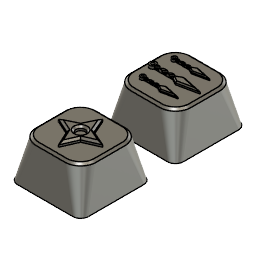
Ninjakeys (Autodesk Fusion 360 design; units mm, degrees)
part number: 2026-03-30-17-35-38-654
Autodesk Fusion 360 part; units mm, degrees
note: some values were not read from the file. Chosen so that the rebuilt part matches the saved one: which face or edge a step refers to.
sketch "Sketch1" plane through (0, 0, 0) normal (0, 1, 0) x (1, 0, 0)
  line L0 (7, -9) -> (-7, -9)
  line L1 (-9, -7) -> (-9, 7)
  line L2 (-7, 9) -> (7, 9)
  line L3 (9, 7) -> (9, -7)
  line L4 (9, -9) -> (-9, 9) construction
  line L5 (-9, -9) -> (9, 9) construction
  arc A0 (-7, 9) -> (-9, 7) centre (-7, 7) ccw
  arc A1 (9, 7) -> (7, 9) centre (7, 7) ccw
  arc A2 (7, -9) -> (9, -7) centre (7, -7) ccw
  arc A3 (-9, -7) -> (-7, -9) centre (-7, -7) ccw
  dimension "d1" = 18
  dimension "d2" = 18
  dimension "d3" = 2
  dimension "d4" = 2
  dimension "d5" = 2
  dimension "d6" = 2
  constraint horizontal L0
  constraint perpendicular L0 L1
  constraint parallel L0 L2
  constraint parallel L1 L3
  constraint coincident L4 origin
  constraint coincident L5 origin
  constraint coincident L4.end L2
  constraint coincident L4.end L1
  constraint tangent L2 A0
  constraint tangent L1 A0
  constraint coincident L5.end L2
  constraint coincident L5.end L3
  constraint tangent L2 A1
  constraint tangent L3 A1
  constraint coincident L4.start L0
  constraint coincident L4.start L3
  constraint tangent L0 A2
  constraint tangent L3 A2
  constraint coincident L5.start L0
  constraint coincident L5.start L1
  constraint tangent L0 A3
  constraint tangent L1 A3
  measures "d1" distance of L4.end L5.end
  measures "d2" distance of L5.start L4.end
  measures "d3" radius of A0
  measures "d4" radius of A1
  measures "d5" radius of A2
  measures "d6" radius of A3
ref_plane "WorkPlane1" through (0, 10, 0) normal (0, 1, 0) x (1, 0, 0)
sketch "Sketch2" plane through (0, 10, 0) normal (0, 1, 0) x (1, 0, 0)
  line L0 (3.5, -7.5) -> (-3.5, -7.5)
  line L1 (-7.5, -3.5) -> (-7.5, 3.5)
  line L2 (-3.5, 7.5) -> (3.5, 7.5)
  line L3 (7.5, 3.5) -> (7.5, -3.5)
  line L4 (7.5, -7.5) -> (-7.5, 7.5) construction
  line L5 (-7.5, -7.5) -> (7.5, 7.5) construction
  arc A0 (-3.5, 7.5) -> (-7.5, 3.5) centre (-3.5, 3.5) ccw
  arc A1 (-7.5, -3.5) -> (-3.5, -7.5) centre (-3.5, -3.5) ccw
  arc A2 (7.5, 3.5) -> (3.5, 7.5) centre (3.5, 3.5) ccw
  arc A3 (3.5, -7.5) -> (7.5, -3.5) centre (3.5, -3.5) ccw
  dimension "d8" = 15
  dimension "d9" = 15
  dimension "d10" = 4
  dimension "d11" = 4
  dimension "d12" = 4
  dimension "d13" = 4
  constraint horizontal L0
  constraint perpendicular L0 L1
  constraint parallel L0 L2
  constraint parallel L1 L3
  constraint coincident L4 origin
  constraint coincident L5 origin
  constraint coincident L4.end L2
  constraint coincident L4.end L1
  constraint tangent L2 A0
  constraint tangent L1 A0
  constraint coincident L5.start L0
  constraint coincident L5.start L1
  constraint tangent L0 A1
  constraint tangent L1 A1
  constraint coincident L5.end L2
  constraint coincident L5.end L3
  constraint tangent L2 A2
  constraint tangent L3 A2
  constraint coincident L4.start L0
  constraint coincident L4.start L3
  constraint tangent L0 A3
  constraint tangent L3 A3
  measures "d8" distance of L4.end L5.end
  measures "d9" distance of L5.start L4.end
  measures "d10" radius of A0
  measures "d11" radius of A1
  measures "d12" radius of A2
  measures "d13" radius of A3
loft "Loft1" add profiles "Sketch1", "Sketch2" section 1 section 2 makes body 1
shell "Shell1" thickness 1 removed faces 1 at (2.3333, 0, 3) on bodies 1
sketch "Sketch4" plane through (0, 9, 0) normal (0, -1, 0) x (1, 0, 0)
  spline S0 degree 3 poles (-3.7981, -6.6388) (-3.9185, -6.6384) (-4.2445, -6.6305) (-4.797, -6.4579) (-4.9562, -6.3904) (-5.4554, -6.1276) (-5.7528, -5.8783) (-6.2352, -5.2918) (-6.4106, -4.9558) (-6.643, -4.1949) (-6.6388, -3.8753) (-6.6388, -2.5029) (-6.6388, -1.6238) (-6.6388, 0.4704) (-6.6388, 1.6711) (-6.6388, 3.2353) (-6.6592, 3.6248) (-6.6079, 4.3124) (-6.5325, 4.6087) (-6.2807, 5.2077) (-6.0878, 5.496) (-5.5896, 6.0247) (-5.2732, 6.2437) (-4.6118, 6.5389) (-4.274, 6.617) (-3.6622, 6.6501) (-3.39, 6.6388) (-2.7262, 6.6388) (-2.3393, 6.6388) (-1.2893, 6.6388) (-0.6369, 6.6388) (1.3044, 6.6388) (2.5692, 6.6388) (3.8951, 6.6388) (4.224, 6.6347) (4.783, 6.4632) (4.9424, 6.3967) (5.4429, 6.1366) (5.7418, 5.8887) (6.2275, 5.3043) (6.4047, 4.9689) (6.6432, 4.2018) (6.6388, 3.8836) (6.6388, 3.4954) (6.6388, 3.373) (6.6388, 1.3089) (6.6388, -0.5696) (6.6388, -2.8908) (6.6471, -3.377) (6.6368, -3.9301) (6.6315, -4.0102) (6.5893, -4.4056) (6.5019, -4.705) (6.2091, -5.3351) (5.9762, -5.6431) (5.4143, -6.1554) (5.0851, -6.3487) (4.3595, -6.61) (4.0322, -6.6388) (2.4883, -6.6388) (1.2237, -6.6388) (0, -6.6388) (-1.2622, -6.6388) (-2.5245, -6.6388) (-3.7902, -6.6388) (-3.794, -6.6388) (-3.7981, -6.6388) knots -2.01973615 -2.01973615 -2.01973615 -2.01973615 -1.98778124 -1.98778124 -1.9735129 -1.9735129 -1.93956421 -1.93956421 -1.90404512 -1.90404512 -1.86164762 -1.86164762 -1.7780832 -1.7780832 -1.65590778 -1.65590778 -1.61360327 -1.61360327 -1.57829605 -1.57829605 -1.53554689 -1.53554689 -1.48489072 -1.48489072 -1.43585563 -1.43585563 -1.39416826 -1.39416826 -1.33065911 -1.33065911 -1.21603599 -1.21603599 -0.97815888 -0.97815888 -0.95834343 -0.95834343 -0.94963949 -0.94963949 -0.92889287 -0.92889287 -0.90717906 -0.90717906 -0.88083394 -0.88083394 -0.86805791 -0.86805791 -0.65819989 -0.65819989 -0.60006747 -0.60006747 -0.58983944 -0.58983944 -0.54756375 -0.54756375 -0.49178961 -0.49178961 -0.43273454 -0.43273454 -0.36711002 -0.36711002 0 0 0 0.37866803 0.37866803 0.37973785 0.37973785 0.37973785 0.37973785
  circle A0 centre (0, 0) radius 2.75
  line L0 (2, -0.585) -> (-2, -0.585)
  line L1 (-2, -0.585) -> (-2, 0.585)
  line L2 (-2, 0.585) -> (2, 0.585)
  line L3 (2, 0.585) -> (2, -0.585)
  line L4 (2, -0.585) -> (-2, 0.585) construction
  line L5 (-2, -0.585) -> (2, 0.585) construction
  line L6 (0.585, -2) -> (-0.585, -2)
  line L7 (-0.585, -2) -> (-0.585, 2)
  line L8 (-0.585, 2) -> (0.585, 2)
  line L9 (0.585, 2) -> (0.585, -2)
  line L10 (0.585, -2) -> (-0.585, 2) construction
  line L11 (-0.585, -2) -> (0.585, 2) construction
  dimension "d15" = 5.5
  dimension "d16" = 4
  dimension "d17" = 1.17
  dimension "d18" = 1.17
  dimension "d19" = 4
  constraint coincident A0.centre origin
  constraint horizontal L0
  constraint perpendicular L0 L1
  constraint parallel L0 L2
  constraint parallel L1 L3
  constraint coincident L4 A0.centre
  constraint coincident L5 A0.centre
  constraint horizontal L6
  constraint perpendicular L6 L7
  constraint parallel L6 L8
  constraint parallel L7 L9
  constraint coincident L10 A0.centre
  constraint coincident L11 A0.centre
  measures "d15" diameter of A0
  measures "d16" distance of L1.end L2.end
  measures "d17" distance of L0.end L1.end
  measures "d18" distance of L7.end L8.end
  measures "d19" distance of L6.end L7.end
extrude "Extrude1" add sketch "Sketch4" along normal blind 6 contours A0 bodies 1
chamfer "Chamfer1" distance 0.5 angle 45 8 edges at (0, 10, 7.5) (6.3284, 10, 6.3284) (7.5, 10, 0) (6.3284, 10, -6.3284) (0, 10, -7.5) (-6.3284, 10, -6.3284) (-7.5, 10, 0) (-6.3284, 10, 6.3284) on bodies 1
sketch "Sketch5" plane through (0, 10, 0) normal (0, 1, 0) x (-1, 0, 0)
  spline S0 degree 3 poles (3.5, -7) (2.6099, -7) (1.7198, -7) (0.1872, -7) (-0.4553, -7) (-1.5919, -7) (-2.0861, -7) (-2.8868, -7) (-3.1934, -7) (-3.5, -7) (-3.7493, -7) (-4.1606, -6.971) (-5.0783, -6.6613) (-5.5771, -6.3727) (-6.3727, -5.5771) (-6.6613, -5.0783) (-6.971, -4.1606) (-7, -3.7493) (-7, -3.5) (-7, -2.6136) (-7, -1.7272) (-7, -0.1967) (-7, 0.4474) (-7, 1.587) (-7, 2.0824) (-7, 2.8853) (-7, 3.1926) (-7, 3.5) (-7, 3.7493) (-6.971, 4.1606) (-6.6613, 5.0783) (-6.3727, 5.5771) (-5.5771, 6.3727) (-5.0783, 6.6613) (-4.1606, 6.971) (-3.7493, 7) (-3.5, 7) (-2.5733, 7) (-1.6466, 7) (-0.0937, 7) (0.5324, 7) (1.6403, 7) (2.1219, 7) (2.9024, 7) (3.2012, 7) (3.5, 7) (3.7493, 7) (4.1606, 6.971) (5.0782, 6.6613) (5.577, 6.3727) (6.3727, 5.5771) (6.6612, 5.0783) (6.971, 4.1607) (7, 3.7493) (7, 3.5) (7, 2.7834) (7, 2.0667) (7, 0.8078) (7, 0.2654) (7, -0.694) (7, -1.1112) (7, -1.8493) (7, -2.1702) (7, -2.7379) (7, -2.9848) (7, -3.3211) (7, -3.4105) (7, -3.5) (7, -3.6826) (6.9856, -3.9508) (6.8461, -4.5753) (6.7186, -4.9307) (6.2507, -5.7279) (5.8485, -6.1497) (5.006, -6.6938) (4.5841, -6.8481) (3.9285, -6.9868) (3.675, -7) (3.5, -7) knots -1 -1 -1 -1 -0.93592515 -0.93592515 -0.88967912 -0.88967912 -0.85410525 -0.85410525 -0.83203638 -0.83203638 -0.83203638 -0.81152729 -0.81152729 -0.79101819 -0.79101819 -0.7705091 -0.7705091 -0.75 -0.75 -0.75 -0.68619367 -0.68619367 -0.63982811 -0.63982811 -0.60416229 -0.60416229 -0.58203638 -0.58203638 -0.58203638 -0.56152729 -0.56152729 -0.54101819 -0.54101819 -0.5205091 -0.5205091 -0.5 -0.5 -0.5 -0.43329126 -0.43329126 -0.3882178 -0.3882178 -0.35354591 -0.35354591 -0.33203638 -0.33203638 -0.33203638 -0.31152789 -0.31152789 -0.29101879 -0.29101879 -0.2705094 -0.2705094 -0.25 -0.25 -0.25 -0.19841298 -0.19841298 -0.15937455 -0.15937455 -0.12934498 -0.12934498 -0.10624531 -0.10624531 -0.08847634 -0.08847634 -0.08203638 -0.08203638 -0.08203638 -0.06701333 -0.06701333 -0.05198965 -0.05198965 -0.03191819 -0.03191819 -0.01439688 -0.01439688 0 0 0 0
  circle A0 centre (5.7, 0) radius 0.4123
  circle A1 centre (5.7, 0) radius 0.8062
  line L0 (-6.3, 0) -> (-1.1, -1.1)
  line L1 (-6.3, 0) -> (-1.1, 1.1)
  line L2 (-1.1, 1.1) -> (-0.9, 0)
  line L3 (-0.9, 0) -> (-1.1, -1.1)
  line L4 (0.3, -0.3) -> (0.3, 0.3429)
  line L5 (0.3, 0.3429) -> (-1.1, 1.1)
  line L6 (4.95, 0.3429) -> (4.95, -0.3)
  line L7 (4.95, -0.3) -> (0.3, -0.3)
  line L8 (-1.1, -1.1) -> (0.3, -0.3)
  line L9 (0.3, 0.3429) -> (4.95, 0.3429)
  line L10 (-6.3, 0) -> (-0.9, 0)
  line L11 (-0.9, 0) -> (0.3, 0.0214)
  line L12 (1.2, -0.3) -> (2.0571, 0.3429)
  line L13 (2.2, -0.3) -> (3.0571, 0.3429)
  line L14 (3.2, -0.3) -> (4.0571, 0.3429)
  line L15 (4.2, -0.3) -> (4.95, 0.3429)
  line L16 (0.4796, -0.3) -> (1.229, 0.3429)
  point P0 (-6.3, 0)
  point P1 (-1.1, -1.1)
  point P2 (-1.1, 1.1)
  point P3 (0.3, -0.3)
  point P4 (0.3, 0.3429)
  point P5 (4.95, -0.3)
  point P6 (4.95, 0.3429)
  point P7 (-0.9, 0)
  point P8 (1, 0.3429)
  point P9 (2.0571, 0.3429)
  point P10 (3.0571, 0.3429)
  point P11 (4.0571, 0.3429)
  point P12 (1.2, -0.3)
  point P13 (2.2, -0.3)
  point P14 (3.2, -0.3)
  point P15 (4.2, -0.3)
  constraint concentric A0 A1
  constraint coincident P0 L0.start
  constraint coincident P1 L0.end
  constraint coincident P2 L1.end
  constraint coincident P7 L2.end
  constraint coincident P3 L4.start
  constraint coincident P4 L4.end
  constraint vertical L4
  constraint coincident P6 L6.start
  constraint coincident P5 L6.end
  constraint parallel L4 L6
  constraint perpendicular L4 L7
  constraint perpendicular L6 L9
  constraint horizontal L10
  constraint midpoint L4 L11.end
  constraint coincident L9 P8
  constraint coincident L9 P9
  constraint coincident L9 P10
  constraint coincident L9 P11
  constraint coincident L7 P12
  constraint coincident L7 P13
  constraint coincident L7 P14
  constraint coincident L7 P15
  constraint coincident P12 L12.start
  constraint coincident P9 L12.end
  constraint coincident P13 L13.start
  constraint coincident P10 L13.end
  constraint parallel L12 L13
  constraint coincident P14 L14.start
  constraint coincident P11 L14.end
  constraint parallel L12 L14
  constraint coincident P15 L15.start
  constraint coincident L7 L16.start
  constraint coincident L9 L16.end
extrude "Extrude2" add sketch "Sketch5" along normal blind 0.7 separate body contours A1 L6 L7 L15 | L7 L9 L13 L14 | L7 L9 L12 L16 | L3 L4 L8 L11 | L2 L4 L5 L11 | L0 L3 L10 | L1 L2 L10 makes body 2 at (-2.4857, 10.2333, -0.0857) makes body 3 at (-1.4857, 10.2333, -0.0857) makes body 4 at (2.8333, 10, 0) makes body 5 at (-4.45, 10.2333, -0.0857)
extrude "Extrude3" add sketch "Sketch5" along normal blind 0.3 separate body contours L7 L9 L14 L15 | L7 L9 L12 L13 | L4 L7 L9 L16 makes body 6 at (-1.819, 10, -0.0857) makes body 7 at (-0.6695, 10, 0.1286) makes body 8 at (-3.819, 10, -0.0857)
extrude "Extrude4" add sketch "Sketch5" along normal blind 0.7 separate body contours A1 L6 picked at (5.0626, -0.0014) makes body 9
chamfer "Chamfer2" distance 0.3 angle 45 4 edges at (3.7, 10.7, -0.55) (0.4, 10.7, -0.7) (3.7, 10.7, 0.55) (0.4, 10.7, 0.7214) on bodies 4
combine "Combine1" operation add target body 4 tool bodies 3 5 7 9 2 6 8
copy_body "CopyPasteBodies1" bodies 4 makes body 10
move_body "Move1" bodies 10 to x (1, 0, 0) y (0, 1, 0) z (0, 0, 1) at (0, 0, -4)
copy_body "CopyPasteBodies2" bodies 4 makes body 11
move_body "Move2" bodies 11 to x (1, 0, 0) y (0, 1, 0) z (0, 0, 1) at (0, 0, 4)
scale "Scale1" factor 0.75 about (-0.3, 10.3, 3.7) bodies 11
scale "Scale2" factor 0.75 about (-0.3, 10.3, -4.3) bodies 10
copy_body "CopyPasteBodies3" bodies 1 makes body 12
move_body "Move3" bodies 12 to x (1, 0, 0) y (0, 1, 0) z (0, 0, 1) at (0, 0, 24)
sketch "Sketch6" plane through (0, 10, 0) normal (0, 1, 0) x (-1, 0, 0)
  spline S0 degree 3 poles (3.5, 17) (2.6099, 17) (1.7198, 17) (0.1872, 17) (-0.4553, 17) (-1.5919, 17) (-2.0861, 17) (-2.8868, 17) (-3.1934, 17) (-3.5, 17) (-3.7493, 17) (-4.1606, 17.029) (-5.0783, 17.3387) (-5.5771, 17.6273) (-6.3727, 18.4229) (-6.6613, 18.9217) (-6.971, 19.8394) (-7, 20.2507) (-7, 20.5) (-7, 21.3864) (-7, 22.2728) (-7, 23.8033) (-7, 24.4474) (-7, 25.587) (-7, 26.0824) (-7, 26.8853) (-7, 27.1926) (-7, 27.5) (-7, 27.7493) (-6.971, 28.1606) (-6.6613, 29.0783) (-6.3727, 29.5771) (-5.5771, 30.3727) (-5.0783, 30.6613) (-4.1606, 30.971) (-3.7493, 31) (-3.5, 31) (-2.5733, 31) (-1.6466, 31) (-0.0937, 31) (0.5324, 31) (1.6403, 31) (2.1219, 31) (2.9024, 31) (3.2012, 31) (3.5, 31) (3.7493, 31) (4.1606, 30.971) (5.0782, 30.6613) (5.577, 30.3727) (6.3727, 29.5771) (6.6612, 29.0783) (6.971, 28.1607) (7, 27.7493) (7, 27.5) (7, 26.7834) (7, 26.0667) (7, 24.8078) (7, 24.2654) (7, 23.306) (7, 22.8888) (7, 22.1507) (7, 21.8298) (7, 21.2621) (7, 21.0152) (7, 20.6789) (7, 20.5895) (7, 20.5) (7, 20.3174) (6.9856, 20.0492) (6.8461, 19.4247) (6.7186, 19.0693) (6.2507, 18.2721) (5.8485, 17.8503) (5.006, 17.3062) (4.5841, 17.1519) (3.9285, 17.0132) (3.675, 17) (3.5, 17) knots -1 -1 -1 -1 -0.93592515 -0.93592515 -0.88967912 -0.88967912 -0.85410525 -0.85410525 -0.83203638 -0.83203638 -0.83203638 -0.81152729 -0.81152729 -0.79101819 -0.79101819 -0.7705091 -0.7705091 -0.75 -0.75 -0.75 -0.68619367 -0.68619367 -0.63982811 -0.63982811 -0.60416229 -0.60416229 -0.58203638 -0.58203638 -0.58203638 -0.56152729 -0.56152729 -0.54101819 -0.54101819 -0.5205091 -0.5205091 -0.5 -0.5 -0.5 -0.43329126 -0.43329126 -0.3882178 -0.3882178 -0.35354591 -0.35354591 -0.33203638 -0.33203638 -0.33203638 -0.31152789 -0.31152789 -0.29101879 -0.29101879 -0.2705094 -0.2705094 -0.25 -0.25 -0.25 -0.19841298 -0.19841298 -0.15937455 -0.15937455 -0.12934498 -0.12934498 -0.10624531 -0.10624531 -0.08847634 -0.08847634 -0.08203638 -0.08203638 -0.08203638 -0.06701333 -0.06701333 -0.05198965 -0.05198965 -0.03191819 -0.03191819 -0.01439688 -0.01439688 0 0 0 0
  circle A0 centre (0, 24) radius 0.8544
  circle A1 centre (0, 24) radius 1.1662
  line L0 (5.6, 24) -> (1.8, 25.7)
  line L1 (1.8, 25.7) -> (0, 29.6)
  line L2 (0, 29.6) -> (-1.7, 25.7)
  line L3 (-1.7, 25.7) -> (-5.6, 24)
  line L4 (-5.6, 24) -> (-1.7, 22.3)
  line L5 (-1.7, 22.3) -> (0, 18.4)
  line L6 (0, 18.4) -> (1.8, 22.2)
  line L7 (1.8, 22.2) -> (5.6, 24)
  line L8 (3.9, 24) -> (1.2, 25.2)
  line L9 (1.2, 25.2) -> (0, 28)
  line L10 (0, 28) -> (-1.2, 25.2)
  line L11 (-1.2, 25.2) -> (-3.9, 24)
  line L12 (-3.9, 24) -> (-5.6, 24)
  line L13 (-3.9, 24) -> (-1.2, 22.8)
  line L14 (-1.2, 22.8) -> (0, 20)
  line L15 (0, 20) -> (0, 18.4)
  line L16 (0, 20) -> (1.2, 22.8)
  line L17 (1.2, 22.8) -> (1.8, 22.2)
  line L18 (1.2, 22.8) -> (3.9, 24)
  line L19 (0, 28) -> (0, 29.6)
  line L20 (3.9, 24) -> (5.6, 24)
  point P0 (1.2, 25.2)
  point P1 (1.2, 22.8)
  point P2 (-1.2, 22.8)
  point P3 (-1.2, 25.2)
  point P4 (-1.7, 25.7)
  point P5 (1.8, 22.2)
  point P6 (1.8, 25.7)
  point P7 (0, 29.6)
  point P8 (-5.6, 24)
  point P9 (0, 18.4)
  point P10 (5.6, 24)
  point P11 (0, 28)
  point P12 (3.9, 24)
  point P13 (0, 20)
  point P14 (-3.9, 24)
  point P15 (-1.7, 22.3)
  constraint concentric A0 A1
  constraint coincident P10 L0.start
  constraint coincident P6 L0.end
  constraint coincident P7 L1.end
  constraint coincident P4 L2.end
  constraint coincident P8 L3.end
  constraint coincident P15 L4.end
  constraint coincident P9 L5.end
  constraint perpendicular L3 L5
  constraint coincident P5 L6.end
  constraint coincident P12 L8.start
  constraint coincident P0 L8.end
  constraint coincident P11 L9.end
  constraint coincident P3 L10.end
  constraint coincident P14 L11.end
  constraint horizontal L12
  constraint coincident P2 L13.end
  constraint coincident P13 L14.end
  constraint vertical L15
  constraint coincident P1 L16.end
  constraint vertical L19
  constraint perpendicular L19 L20
extrude "Extrude5" add sketch "Sketch6" along normal blind 1 separate body contours L0 L1 L8 L9 L19 L20 | L7 L17 L18 L20 | L6 L15 L16 L17 | L8 L9 L10 L11 L13 L14 L16 L18 | L2 L3 L10 L11 L12 L19 | L4 L5 L12 L13 L14 L15 makes body 13
chamfer "Chamfer3" distance 0.5 angle 45 1 faces at (-2.8554, 11, 23.4) on bodies 13
